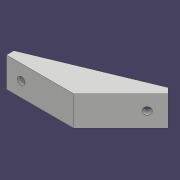
# Autodesk Inventor part: L Bracket Small
Saved by Autodesk Inventor 2017 SP1 (Build 210196100, 196)
## iProperties
Created: 2018-05-02
Part Number: L Bracket Small
Material: Generic
Document SubType Name: Modeling
Designer: Zach
Density: 1 g/cm^3
Appearance: Default
Author: Zach
Autodesk Inventor part; units mm, degrees
ref_plane "YZ Plane" through (0, 0, 0) normal (1, 0, 0) x (0, 1, 0)
ref_plane "XZ Plane" through (0, 0, 0) normal (0, 1, 0) x (-1, 0, 0)
ref_plane "XY Plane" through (0, 0, 0) normal (0, 0, 1) x (1, 0, 0)
sketch "Sketch6" plane through (0, 0, 0) normal (0, 0, 1) x (1, 0, 0)
  line L0 (0, 0) -> (45, 0)
  line L1 (45, 0) -> (76.8198, 31.8198)
  line L2 (76.8198, 31.8198) -> (73.2843, 35.3553)
  line L3 (0, 0) -> (0, 5)
  line L4 (0, 5) -> (42.9289, 5)
  line L5 (42.9289, 5) -> (73.2843, 35.3553)
  dimension "d19" = 45
  dimension "d20" = 45
  dimension "d21" = 135
  dimension "d22" = 5
  dimension "d23" = 5
  constraints: 12 end point, 2 horizontal, 2 perpendicular, 1 vertical
  measures "d19" distance of L0.start L0.end
  measures "d20" distance of L0.end L1.end
  measures "d21" angle of L1 L0
  measures "d22" distance of L1.end L2.end
  measures "d23" distance of L0.start L3.end
extrude "Extrusion6" add sketch "Sketch6" along normal blind 20
sketch "Sketch7" plane through (0, 0, 20) normal (0, 0, 1) x (1, 0, 0)
  line L0 (42.9289, 5) -> (0, 5) projected
  line L1 (76.8198, 31.8198) -> (73.2843, 35.3553) projected
  line L2 (0, 5) -> (73.2843, 35.3553)
  line L3 (73.2843, 35.3553) -> (42.9289, 5) projected
  point P0 (0, 0)
  constraints: 2 end point
extrude "Extrusion7" add sketch "Sketch7" against normal blind 2
sketch "Sketch8" plane through (0, 0, 0) normal (0, 0, -1) x (-1, 0, 0)
  line L0 (0, 5) -> (-42.9289, 5) projected
  line L1 (0, 5) -> (-73.2843, 35.3553) projected
  line L2 (-42.9289, 5) -> (-73.2843, 35.3553) projected
  point P0 (0, 0)
extrude "Extrusion8" add sketch "Sketch8" against normal blind 2
sketch "Sketch9" plane through (0, 5, 18) normal (0, 1, 0) x (1, 0, 0)
  circle A0 centre (10, 8) radius 2.5
  line L0 (0, 16) -> (0, 0) projected
  point P0 (0, 18)
  point P1 (0, 8)
  dimension "d30" = 5
  dimension "d31" = 10
  constraints: 1 centre point, 1 horizontal alignment, 1 midpoint
  measures "d30" diameter of A0
  measures "d31" distance of point (0, 8) A0.centre
extrude "Extrusion9" cut sketch "Sketch9" against normal through all
sketch "Sketch10" plane through (42.9289, 5, 2) normal (-0.7071, 0.7071, 0) x (-0.7071, -0.7071, 0)
  circle A0 centre (-32.9289, 8) radius 2.5
  line L0 (-42.9289, 0) -> (-42.9289, 16) projected
  point P0 (33.8909, -2)
  point P1 (-42.9289, 8)
  dimension "d34" = 5
  dimension "d35" = 10
  constraints: 1 centre point, 1 horizontal alignment, 1 midpoint
  measures "d34" diameter of A0
  measures "d35" distance from line of L0 A0.centre
extrude "Extrusion10" cut sketch "Sketch10" against normal through all
body "Solid2"
